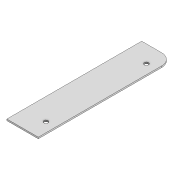
# Autodesk Inventor part: sidewall inside
Saved by Autodesk Inventor 2020 (Build 240168000, 168)
## iProperties
Created: 2020-03-01
Part Number: sidewall inside
Material: Generic
Document SubType Name: Modeling
Designer: ball
Density: 1 g/cm^3
Appearance: Default
Author: ball
Autodesk Inventor part; units mm, degrees
ref_plane "YZ Plane" through (0, 0, 0) normal (1, 0, 0) x (0, 1, 0)
ref_plane "XZ Plane" through (0, 0, 0) normal (0, 1, 0) x (-1, 0, 0)
ref_plane "XY Plane" through (0, 0, 0) normal (0, 0, 1) x (1, 0, 0)
sketch "Sketch1" plane through (0, 0, 0) normal (0, 1, 0) x (-1, 0, 0)
  line L0 (0, 0) -> (104.9602, 0)
  line L1 (104.9602, 0) -> (104.9602, -450.85)
  line L2 (104.9602, -450.85) -> (38.1, -450.85)
  line L3 (0, -412.75) -> (0, 0)
  arc A0 (0, -412.75) -> (38.1, -450.85) centre (38.1, -412.75) ccw
  line L4 (38.1, -412.75) -> (38.1, -450.85) construction
  line L5 (38.1, -412.75) -> (76.2, -412.75) construction
  dimension "d1" = 450.85
  dimension "d5" = 38.1
  dimension "d6" = 90
  dimension "d7" = 104.9602
  dimension "d8" = 38.1
  constraints: 12 end point, 2 horizontal, 2 parallel, 2 perpendicular, 2 point on circle, 1 centre point, 1 coincident
  measures "d1" distance of L0.end L1.end
  measures "d5" radius of A0
  measures "d6" angle of L4 L5
  measures "d7" distance between parallel lines of L3 L1
  measures "d8" distance from line of L3 point (38.1, -412.75)
extrude "Extrusion1" add sketch "Sketch1" along normal blind 5
sketch "Sketch2" plane through (0, 5, 0) normal (0, 1, 0) x (1, 0, 0)
  circle A0 centre (-31.75, 57.3786) radius 7.1016
  line L0 (-104.9602, 0) -> (0, 0) projected
  line L1 (0, 0) -> (0, 412.75) projected
  circle A1 centre (-31.75, 393.4714) radius 7.1016
  circle A2 centre (-9.8044, 14.0462) radius 1.7
  circle A3 centre (-9.8044, 24.0462) radius 1.7
  circle A4 centre (-19.8044, 14.0462) radius 1.7
  circle A5 centre (-19.8044, 24.0462) radius 1.7
  circle A6 centre (-69.342, 14.0462) radius 1.7
  circle A7 centre (-79.342, 14.0462) radius 1.7
  circle A8 centre (-69.342, 24.0462) radius 1.7
  circle A9 centre (-79.342, 24.0462) radius 1.7
  circle A10 centre (-10.16, 76.2) radius 1.778
  circle A11 centre (-10.16, 88.9) radius 1.778
  circle A12 centre (-10.16, 101.6) radius 1.778
  circle A13 centre (-10.16, 114.3) radius 1.778
  circle A14 centre (-10.16, 127) radius 1.778
  circle A15 centre (-10.16, 139.7) radius 1.778
  circle A16 centre (-10.16, 152.4) radius 1.778
  circle A17 centre (-10.16, 165.1) radius 1.778
  circle A18 centre (-10.16, 177.8) radius 1.778
  circle A19 centre (-10.16, 190.5) radius 1.778
  circle A20 centre (-10.16, 203.2) radius 1.778
  circle A21 centre (-10.16, 215.9) radius 1.778
  circle A22 centre (-10.16, 228.6) radius 1.778
  circle A23 centre (-10.16, 241.3) radius 1.778
  circle A24 centre (-10.16, 254) radius 1.778
  circle A25 centre (-10.16, 266.7) radius 1.778
  circle A26 centre (-10.16, 279.4) radius 1.778
  circle A27 centre (-10.16, 292.1) radius 1.778
  circle A28 centre (-10.16, 304.8) radius 1.778
  circle A29 centre (-10.16, 317.5) radius 1.778
  circle A30 centre (-10.16, 330.2) radius 1.778
  circle A31 centre (-10.16, 342.9) radius 1.778
  circle A32 centre (-10.16, 355.6) radius 1.778
  circle A33 centre (-22.86, 76.2) radius 1.778
  circle A34 centre (-22.86, 88.9) radius 1.778
  circle A35 centre (-22.86, 101.6) radius 1.778
  circle A36 centre (-22.86, 114.3) radius 1.778
  circle A37 centre (-22.86, 127) radius 1.778
  circle A38 centre (-22.86, 139.7) radius 1.778
  circle A39 centre (-22.86, 152.4) radius 1.778
  circle A40 centre (-22.86, 165.1) radius 1.778
  circle A41 centre (-22.86, 177.8) radius 1.778
  circle A42 centre (-22.86, 190.5) radius 1.778
  circle A43 centre (-22.86, 203.2) radius 1.778
  circle A44 centre (-22.86, 215.9) radius 1.778
  circle A45 centre (-22.86, 228.6) radius 1.778
  circle A46 centre (-22.86, 241.3) radius 1.778
  circle A47 centre (-22.86, 254) radius 1.778
  circle A48 centre (-22.86, 266.7) radius 1.778
  circle A49 centre (-22.86, 279.4) radius 1.778
  circle A50 centre (-22.86, 292.1) radius 1.778
  circle A51 centre (-22.86, 304.8) radius 1.778
  circle A52 centre (-22.86, 317.5) radius 1.778
  circle A53 centre (-22.86, 330.2) radius 1.778
  circle A54 centre (-22.86, 342.9) radius 1.778
  circle A55 centre (-22.86, 355.6) radius 1.778
  circle A56 centre (-35.56, 76.2) radius 1.778
  circle A57 centre (-35.56, 88.9) radius 1.778
  circle A58 centre (-35.56, 101.6) radius 1.778
  circle A59 centre (-35.56, 114.3) radius 1.778
  circle A60 centre (-35.56, 127) radius 1.778
  circle A61 centre (-35.56, 139.7) radius 1.778
  circle A62 centre (-35.56, 152.4) radius 1.778
  circle A63 centre (-35.56, 165.1) radius 1.778
  circle A64 centre (-35.56, 177.8) radius 1.778
  circle A65 centre (-35.56, 190.5) radius 1.778
  circle A66 centre (-35.56, 203.2) radius 1.778
  circle A67 centre (-35.56, 215.9) radius 1.778
  circle A68 centre (-35.56, 228.6) radius 1.778
  circle A69 centre (-35.56, 241.3) radius 1.778
  circle A70 centre (-35.56, 254) radius 1.778
  circle A71 centre (-35.56, 266.7) radius 1.778
  circle A72 centre (-35.56, 279.4) radius 1.778
  circle A73 centre (-35.56, 292.1) radius 1.778
  circle A74 centre (-35.56, 304.8) radius 1.778
  circle A75 centre (-35.56, 317.5) radius 1.778
  circle A76 centre (-35.56, 330.2) radius 1.778
  circle A77 centre (-35.56, 342.9) radius 1.778
  circle A78 centre (-35.56, 355.6) radius 1.778
  circle A79 centre (-48.26, 76.2) radius 1.778
  circle A80 centre (-48.26, 88.9) radius 1.778
  circle A81 centre (-48.26, 101.6) radius 1.778
  circle A82 centre (-48.26, 114.3) radius 1.778
  circle A83 centre (-48.26, 127) radius 1.778
  circle A84 centre (-48.26, 139.7) radius 1.778
  circle A85 centre (-48.26, 152.4) radius 1.778
  circle A86 centre (-48.26, 165.1) radius 1.778
  circle A87 centre (-48.26, 177.8) radius 1.778
  circle A88 centre (-48.26, 190.5) radius 1.778
  circle A89 centre (-48.26, 203.2) radius 1.778
  circle A90 centre (-48.26, 215.9) radius 1.778
  circle A91 centre (-48.26, 228.6) radius 1.778
  circle A92 centre (-48.26, 241.3) radius 1.778
  circle A93 centre (-48.26, 254) radius 1.778
  circle A94 centre (-48.26, 266.7) radius 1.778
  circle A95 centre (-48.26, 279.4) radius 1.778
  circle A96 centre (-48.26, 292.1) radius 1.778
  circle A97 centre (-48.26, 304.8) radius 1.778
  circle A98 centre (-48.26, 317.5) radius 1.778
  circle A99 centre (-48.26, 330.2) radius 1.778
  circle A100 centre (-48.26, 342.9) radius 1.778
  circle A101 centre (-48.26, 355.6) radius 1.778
  circle A102 centre (-60.96, 76.2) radius 1.778
  circle A103 centre (-60.96, 88.9) radius 1.778
  circle A104 centre (-60.96, 101.6) radius 1.778
  circle A105 centre (-60.96, 114.3) radius 1.778
  circle A106 centre (-60.96, 127) radius 1.778
  circle A107 centre (-60.96, 139.7) radius 1.778
  circle A108 centre (-60.96, 152.4) radius 1.778
  circle A109 centre (-60.96, 165.1) radius 1.778
  circle A110 centre (-60.96, 177.8) radius 1.778
  circle A111 centre (-60.96, 190.5) radius 1.778
  circle A112 centre (-60.96, 203.2) radius 1.778
  circle A113 centre (-60.96, 215.9) radius 1.778
  circle A114 centre (-60.96, 228.6) radius 1.778
  circle A115 centre (-60.96, 241.3) radius 1.778
  circle A116 centre (-60.96, 254) radius 1.778
  circle A117 centre (-60.96, 266.7) radius 1.778
  circle A118 centre (-60.96, 279.4) radius 1.778
  circle A119 centre (-60.96, 292.1) radius 1.778
  circle A120 centre (-60.96, 304.8) radius 1.778
  circle A121 centre (-60.96, 317.5) radius 1.778
  circle A122 centre (-60.96, 330.2) radius 1.778
  circle A123 centre (-60.96, 342.9) radius 1.778
  circle A124 centre (-60.96, 355.6) radius 1.778
  circle A125 centre (-73.66, 76.2) radius 1.778
  circle A126 centre (-73.66, 88.9) radius 1.778
  circle A127 centre (-73.66, 101.6) radius 1.778
  circle A128 centre (-73.66, 114.3) radius 1.778
  circle A129 centre (-73.66, 127) radius 1.778
  circle A130 centre (-73.66, 139.7) radius 1.778
  circle A131 centre (-73.66, 152.4) radius 1.778
  circle A132 centre (-73.66, 165.1) radius 1.778
  circle A133 centre (-73.66, 177.8) radius 1.778
  circle A134 centre (-73.66, 190.5) radius 1.778
  circle A135 centre (-73.66, 203.2) radius 1.778
  circle A136 centre (-73.66, 215.9) radius 1.778
  circle A137 centre (-73.66, 228.6) radius 1.778
  circle A138 centre (-73.66, 241.3) radius 1.778
  circle A139 centre (-73.66, 254) radius 1.778
  circle A140 centre (-73.66, 266.7) radius 1.778
  circle A141 centre (-73.66, 279.4) radius 1.778
  circle A142 centre (-73.66, 292.1) radius 1.778
  circle A143 centre (-73.66, 304.8) radius 1.778
  circle A144 centre (-73.66, 317.5) radius 1.778
  circle A145 centre (-73.66, 330.2) radius 1.778
  circle A146 centre (-73.66, 342.9) radius 1.778
  circle A147 centre (-73.66, 355.6) radius 1.778
  circle A148 centre (-86.36, 76.2) radius 1.778
  circle A149 centre (-86.36, 88.9) radius 1.778
  circle A150 centre (-86.36, 101.6) radius 1.778
  circle A151 centre (-86.36, 114.3) radius 1.778
  circle A152 centre (-86.36, 127) radius 1.778
  circle A153 centre (-86.36, 139.7) radius 1.778
  circle A154 centre (-86.36, 152.4) radius 1.778
  circle A155 centre (-86.36, 165.1) radius 1.778
  circle A156 centre (-86.36, 177.8) radius 1.778
  circle A157 centre (-86.36, 190.5) radius 1.778
  circle A158 centre (-86.36, 203.2) radius 1.778
  circle A159 centre (-86.36, 215.9) radius 1.778
  circle A160 centre (-86.36, 228.6) radius 1.778
  circle A161 centre (-86.36, 241.3) radius 1.778
  circle A162 centre (-86.36, 254) radius 1.778
  circle A163 centre (-86.36, 266.7) radius 1.778
  circle A164 centre (-86.36, 279.4) radius 1.778
  circle A165 centre (-86.36, 292.1) radius 1.778
  circle A166 centre (-86.36, 304.8) radius 1.778
  circle A167 centre (-86.36, 317.5) radius 1.778
  circle A168 centre (-86.36, 330.2) radius 1.778
  circle A169 centre (-86.36, 342.9) radius 1.778
  circle A170 centre (-86.36, 355.6) radius 1.778
  circle A171 centre (-9.8044, 344.2462) radius 1.7
  circle A172 centre (-9.8044, 354.2462) radius 1.7
  circle A173 centre (-19.8044, 344.2462) radius 1.7
  circle A174 centre (-19.8044, 354.2462) radius 1.7
  circle A175 centre (-6.35, 6.35) radius 2.25
  line L2 (-19.8044, 24.0462) -> (-9.8044, 14.0462) construction
  line L3 (-9.8044, 24.0462) -> (-19.8044, 14.0462) construction
  line L4 (-22.3044, 26.5462) -> (-7.3044, 26.5462) construction
  line L5 (-7.3044, 26.5462) -> (-7.3044, 11.5462) construction
  line L6 (-7.3044, 11.5462) -> (-22.3044, 11.5462) construction
  line L7 (-22.3044, 11.5462) -> (-22.3044, 26.5462) construction
  line L8 (-22.3044, 26.5462) -> (-7.3044, 11.5462) construction
  line L9 (-7.3044, 26.5462) -> (-22.3044, 11.5462) construction
  point P0 (-14.8044, 19.0462)
  dimension "bearingHole" = 14.2032
  dimension "d12" = 57.3786
  dimension "d13" = 31.75
  dimension "d14" = 14.2032
  dimension "d15" = 31.75
  dimension "d16" = 336.0928
  dimension "M3Clearance" = 3.4
  dimension "d20" = 14.0462
  dimension "d21" = 9.8044
  dimension "d24" = 10
  dimension "d27" = 10
  dimension "d30" = 3.4
  dimension "d31" = 14.0462
  dimension "d32" = 69.342
  dimension "d42" = 10
  dimension "d45" = 10
  dimension "Number6Clearance" = 3.556
  dimension "d49" = 10.16
  dimension "d50" = 76.2
  dimension "d53" = 12.7
  dimension "d56" = 12.7
  dimension "d59" = 3.4
  dimension "d60" = 9.8044
  dimension "d61" = 344.2462
  dimension "d64" = 10
  dimension "d67" = 10
  dimension "d70" = 4.5
  dimension "d71" = 6.35
  dimension "d72" = 6.35
  dimension "d73" = 15
  dimension "d74" = 15
  constraints: 176 centre point, 16 end point, 5 horizontal, 4 vertical, 3 midpoint, 2 parallel, 1 perpendicular, 338 other
  measures "bearingHole" diameter of A0
  measures "d12" distance from line of L0 A0.centre
  measures "d13" distance from line of L1 A0.centre
  measures "d14" diameter of A1
  measures "d15" distance from line of L1 A1.centre
  measures "d16" distance of A0.centre A1.centre
  measures "M3Clearance" diameter of A2
  measures "d20" distance from line of L0 L2.end
  measures "d21" distance from line of L1 L2.end
  measures "d24" distance of L2.end L3.start
  measures "d27" distance of L2.end L3.end
  measures "d30" diameter of A6
  measures "d31" distance from line of L0 A6.centre
  measures "d32" distance from line of L1 A6.centre
  measures "d42" distance of A6.centre A7.centre
  measures "d45" distance of A6.centre A8.centre
  measures "Number6Clearance" diameter of A10
  measures "d49" distance from line of L1 A10.centre
  measures "d50" distance from line of L0 A10.centre
  measures "d53" distance of A10.centre A11.centre
  measures "d56" distance of A10.centre A33.centre
  measures "d59" diameter of A171
  measures "d60" distance from line of L1 A171.centre
  measures "d61" distance from line of L0 A171.centre
  measures "d64" distance of A171.centre A172.centre
  measures "d67" distance of A171.centre A173.centre
  measures "d70" diameter of A175
  measures "d71" distance from line of L1 A175.centre
  measures "d72" distance from line of L0 A175.centre
  measures "d73" distance of L5.end L6.end
  measures "d74" distance of L4.end L5.end
extrude "Extrusion2" cut sketch "Sketch2" against normal through all contours A0 | A1
equation "\"d14\" = bearingHole"
equation "\"d15\" = d13"
equation "\"d30\" = M3Clearance"
equation "\"d31\" = d20"
equation "\"d59\" = M3Clearance"
equation "\"d60\" = d21"
body "Solid1"
